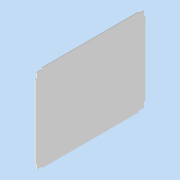
# Autodesk Inventor part: Acrly_Wand_1
Saved by Autodesk Inventor 2022 (Build 260153000, 153)
## iProperties
Created: 2021-12-15
Part Number: Acrly_Wand_1
Material: Generic
Document SubType Name: Modeling
Designer: Fabijansven
Density: 1 g/cm^3
Appearance: Default
Author: Fabijansven
Autodesk Inventor part; units mm, degrees
ref_plane "YZ Plane" through (0, 0, 0) normal (1, 0, 0) x (0, 1, 0)
ref_plane "XZ Plane" through (0, 0, 0) normal (0, 1, 0) x (-1, 0, 0)
ref_plane "XY Plane" through (0, 0, 0) normal (0, 0, 1) x (1, 0, 0)
sketch "Sketch1" plane through (0, 0, 0) normal (1, 0, 0) x (0, 1, 0)
  line L0 (0, 0) -> (522, 0)
  line L1 (522, 0) -> (522, -662)
  line L2 (522, -662) -> (0, -662)
  line L3 (0, -662) -> (0, 0)
  line L4 (522, 0) -> (514, 0)
  line L5 (514, 0) -> (514, -40)
  line L6 (514, -40) -> (522, -40)
  line L7 (522, -40) -> (522, 0)
  line L8 (522, 0) -> (482, 0)
  line L9 (482, 0) -> (482, -8)
  line L10 (482, -8) -> (522, -8)
  line L11 (522, -8) -> (522, 0)
  line L12 (856.5319, -331) -> (-65.1606, -331) construction
  line L13 (261, 165.682) -> (261, -1074.2454) construction
  line L14 (522, -662) -> (514, -662)
  line L15 (514, -662) -> (514, -622)
  line L16 (514, -622) -> (522, -622)
  line L17 (522, -622) -> (522, -662)
  line L18 (522, -662) -> (482, -662)
  line L19 (482, -662) -> (482, -654)
  line L20 (482, -654) -> (522, -654)
  line L21 (522, -654) -> (522, -662)
  line L22 (0, 0) -> (0, -662)
  line L23 (0, 0) -> (8, 0)
  line L24 (8, 0) -> (8, -40)
  line L25 (8, -40) -> (0, -40)
  line L26 (0, -40) -> (0, 0)
  line L27 (0, 0) -> (40, 0)
  line L28 (40, 0) -> (40, -8)
  line L29 (40, -8) -> (0, -8)
  line L30 (0, -8) -> (0, 0)
  line L31 (8, -622) -> (0, -622)
  line L32 (40, -654) -> (0, -654)
  line L33 (0, -662) -> (8, -662)
  line L34 (8, -662) -> (8, -622)
  line L35 (0, -622) -> (0, -662)
  line L36 (0, -662) -> (40, -662)
  line L37 (40, -662) -> (40, -654)
  line L38 (0, -654) -> (0, -662)
  point P0 (482, -662)
  point P1 (514, -654)
  point P2 (522, -622)
  point P3 (522, -40)
  point P4 (514, -8)
  point P5 (482, 0)
  point P6 (40, 0)
  point P7 (8, -8)
  point P8 (0, -40)
  point P9 (0, -622)
  point P10 (8, -654)
  dimension "d0" = 522
  dimension "d1" = 662
  dimension "d2" = 40
  dimension "d3" = 40
  dimension "d4" = 8
  dimension "d5" = 8
  dimension "d6" = 331
  dimension "d7" = 261
  constraints: 78 end point, 18 symmetric about line, 6 parallel, 4 horizontal, 3 perpendicular, 1 vertical
  measures "d0" distance of L1.end L2.end
  measures "d1" distance of L0.end L1.end
  measures "d2" distance of L4.end L5.end
  measures "d3" distance of L9.end L10.end
  measures "d4" distance of L8.end L9.end
  measures "d5" distance of L5.end L6.end
  measures "d6" distance between parallel lines of L0 L12
  measures "d7" distance between parallel lines of L3 L13
extrude "Extrusion1" add sketch "Sketch1" along normal blind 5 contours L0 L9 L10 L5 L6 L1 L16 L15 L20 L19 L2 L37 L32 L34 L31 L3 L25 L24 L29 L28
equation "\"d6\" = 0.5 * d1"
equation "\"d7\" = 0.5 * d0"
body "Solid1"
